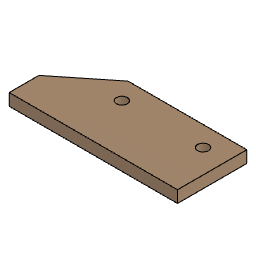
Z Endswitch plate (Autodesk Fusion 360 design; units mm, degrees)
Autodesk Fusion 360 part; units mm, degrees
sketch "Z Endswitch plate" plane through (0, 0, 0) normal (0, 0, 1) x (1, 0, 0)
  line L0 (18, -15) -> (18, 20)
  circle A0 centre (6, 9.9027) radius 2.75
  line L1 (-67, 20) -> (-67, -15)
  line L2 (-67, -15) -> (18, -15)
  line L3 (-42, 20) -> (-67, 0)
  circle A1 centre (-35, 9.9027) radius 2.75
  line L4 (18, 20) -> (-67, 20)
  line L5 (18, 9.9027) -> (-67, 9.9027) construction
  dimension "d2" = 85
  dimension "d3" = 5.5
  dimension "d4" = 5.5
  dimension "d7" = 25
  dimension "d8" = 20
  dimension "d9" = 15
  dimension "d10" = 18
  dimension "d11" = 6
  dimension "d12" = 35
  constraint horizontal L2
  constraint vertical L0
  constraint horizontal L4
  constraint vertical L1
  constraint coincident L5.start L0
  constraint coincident L5.end L1
  constraint perpendicular L1 L5
  constraint coincident A0.centre L5
  constraint coincident A1.centre L5
  constraint coincident L3.start L4
  constraint coincident L3.end L1
  measures "d2" distance of L0.start L1.end
  measures "d3" diameter of A0
  measures "d4" diameter of A1
  measures "d7" distance of L3.start L1
  measures "d8" distance of origin L4
  measures "d9" distance of origin L2
  measures "d10" distance of origin L0
  measures "d11" horizontal distance of origin A0.centre
  measures "d12" horizontal distance of origin A1.centre
extrude "Extrude1" add sketch "Z Endswitch plate" along normal blind 6 contours L0 L1 L2 L3 L4
named bodies: "Z Endswitch plate"
